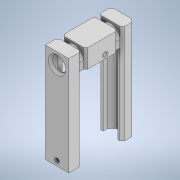
# Autodesk Inventor part: Magazin
Saved by Autodesk Inventor 2021 (Build 250183000, 183)
## iProperties
Created: 2024-05-14
Part Number: Magazin
Material: Generic
Document SubType Name: Modeling
Designer: Lukas
Density: 1 g/cm^3
Appearance: Default
Author: Lukas
Autodesk Inventor part; units mm, degrees
ref_plane "YZ Plane" through (0, 0, 0) normal (1, 0, 0) x (0, 1, 0)
ref_plane "XZ Plane" through (0, 0, 0) normal (0, 1, 0) x (-1, 0, 0)
ref_plane "XY Plane" through (0, 0, 0) normal (0, 0, 1) x (1, 0, 0)
sketch "Sketch1" plane through (0, 0, 0) normal (0, 0, 1) x (1, 0, 0)
  circle A0 centre (0, 0) radius 5
  line L0 (-8, 0) -> (-8, -60)
  line L1 (-8, -60) -> (8, -60)
  line L2 (8, -60) -> (8, 0)
  line L3 (8, 0) -> (8, 8)
  line L4 (8, 8) -> (-8, 8)
  line L5 (-8, 8) -> (-8, 0)
  point P0 (0, 8)
  dimension "d0" = 10
  dimension "d3" = 60
  dimension "d4" = 16
  dimension "d68" = 8
  constraints: 12 end point, 3 perpendicular, 2 horizontal alignment, 2 vertical, 1 centre point, 1 coincident, 1 collinear, 1 midpoint, 1 vertical alignment
  measures "d0" diameter of A0
  measures "d3" distance of L1.end L2.end
  measures "d4" distance between parallel lines of L2 L0
  measures "d68" distance of L4.end L0.start
extrude "Extrusion1" add sketch "Sketch1" along normal mid plane 45
sketch "Sketch3" plane through (-8, -60, -22.5) normal (0, -1, 0) x (1, 0, 0)
  line L0 (13, 45) -> (13, 0) projected
  line L1 (13, 5.5) -> (10, 2.5)
  line L2 (10, 2.5) -> (6, 2.5)
  line L3 (6, 2.5) -> (3, 5.5)
  line L4 (3, 45) -> (3, 0) projected
  line L5 (13, 39.5) -> (10, 42.5)
  line L6 (10, 42.5) -> (6, 42.5)
  line L7 (6, 42.5) -> (3, 39.5)
  line L8 (16, 0) -> (0, 0) projected
  point P0 (8, 22.5)
  point P1 (8, 0)
  dimension "d19" = 4
  dimension "d20" = 3
  dimension "d21" = 40
  dimension "d54" = 20
  constraints: 12 end point, 4 point on line, 3 equal length, 2 horizontal alignment, 2 parallel, 1 perpendicular, 2 other
  measures "d19" distance of L1.end L2.end
  measures "d20" distance from line of L2 L1.start
  measures "d21" distance between parallel lines of L2 L6
  measures "d54" distance from line of point (8, 22.5) L2
extrude "Extrusion3" cut sketch "Sketch3" against normal blind 60 contours L0 L1 L2 L3 L4 L7 L6 L5
sketch "Sketch4" plane through (-8, -60, -22.5) normal (0, -1, 0) x (1, 0, 0)
  line L0 (16, 0) -> (0, 0) projected
  line L1 (14.2, 0) -> (16, 1.8)
  line L2 (16, 0) -> (16, 45) projected
  line L3 (1.8, 0) -> (0, 1.8)
  line L4 (0, 0) -> (0, 45) projected
  line L5 (13, 5.5) -> (10, 2.5) projected
  point P0 (8, 22.5)
  dimension "d35" = 1.8
  constraints: 4 end point, 2 point on line, 1 horizontal alignment, 1 parallel, 1 perpendicular, 3 other
  measures "d35" horizontal distance of L1.start L1.end
extrude "Extrusion4" cut sketch "Sketch4" against normal through all
ref_plane "Work Plane3" through (0, 0, -2.4) normal (0, 0, 1) x (1, 0, 0)
sketch "Sketch5" plane through (0, 0, -2.4) normal (0, 0, 1) x (1, 0, 0)
  line L0 (8, -60) -> (8, 8) projected
  line L1 (8, -1) -> (8, -4)
  arc A0 (8, -1) -> (8, -4) centre (9.125, -2.5) ccw
  line L2 (9.125, -2.5) -> (9.125, -1.8268)
  point P0 (0, 0)
  point P1 (8, 0)
  point P2 (8, -1)
  dimension "d42" = 3
  dimension "d43" = 0.75
  dimension "d44" = 2.5
  dimension "d45" = 8
  constraints: 4 end point, 2 point on circle, 2 vertical, 1 centre point
  measures "d42" distance of L1.start L1.end
  measures "d43" distance edge to line of A0 L1
  measures "d44" vertical distance of point (0, 0) L2.start
  measures "d45" horizontal distance of point (0, 0) L1.start
revolve "Revolution1" cut sketch "Sketch5" angle 360 about axis through (9.125, -2.5, -2.4) along (0, 1, 0)
fillet "Fillet1" radius 1 2 edges at (8, -2.5, -0.9) (8, -2.5, -3.9)
mirror "Mirror1" about plane through (0, 0, 0) normal (1, 0, 0) of "Revolution1", "Fillet1"
ref_plane "Work Plane2" through (0, 0, -12.5) normal (0, 0, -1) x (-1, 0, 0)
sketch "Sketch6" plane through (0, 0, -12.5) normal (0, 0, -1) x (-1, 0, 0)
  line L0 (-8, -60) -> (-8, 8) projected
  line L1 (8, 8) -> (8, -60) projected
  arc A0 (6.5, 0) -> (-6.5, 0) centre (0, 0) ccw
  line L2 (6.5, 0) -> (6.5, -5)
  line L3 (6.5, -5) -> (5, -5)
  line L4 (5, -60) -> (5, 0) projected
  line L5 (-6.5, 0) -> (-6.5, -5)
  line L6 (-6.5, -5) -> (-5, -5)
  line L7 (-5, -60) -> (-5, 0) projected
  line L8 (8, -60) -> (-8, -60) projected
  line L9 (-8, 8) -> (8, 8) projected
  circle A1 centre (0, 0) radius 5 projected
  point P0 (-8, 0)
  point P1 (8, 0)
  dimension "d50" = 5
  dimension "d69" = 1.5
  constraints: 8 end point, 4 point on line, 2 perpendicular, 2 point on circle, 2 tangent, 1 centre point, 1 concentric, 1 vertical
  measures "d50" distance from line of point (0, 0) L6
  measures "d69" distance of L5.end L6.end
extrude "Extrusion5" cut sketch "Sketch6" against normal mid plane 3 contours L0 L9 L1 L8 L4 L3 L2 A0 L5 L6 L7
chamfer "Chamfer4" distance 1.5 angle 45 4 edges at (-8, -26, -11) (8, -26, -11) (-8, -26, -14) (8, -26, -14)
mirror "Mirror2" about plane through (0, 0, 0) normal (0, 0, 1) of "Extrusion5", "Chamfer4"
chamfer "Chamfer5" distance 1 distance2 2 1 edges at (-5, 0, 22.5) measured on face at (-5.5, 0, 22.5)
sketch "Sketch7" plane through (0, 0, 22.5) normal (0, 0, 1) x (1, 0, 0)
  circle A0 centre (0, -56.6) radius 1.6
  line L0 (-8, -60) -> (8, -60) projected
  point P0 (0, 0)
  point P1 (0, -60)
  dimension "d58" = 3.4
  dimension "d59" = 3.2
  constraints: 1 centre point, 1 midpoint, 1 vertical alignment
  measures "d58" distance from line of L0 A0.centre
  measures "d59" diameter of A0
extrude "Extrusion6" cut sketch "Sketch7" against normal through all
sketch "Sketch9" plane through (-6.5, -60, -11) normal (0, -1, 0) x (1, 0, 0)
  line L0 (13, 22) -> (14.5, 20.5) projected
  line L1 (13, 22) -> (11.5, 22) projected
  line L2 (11.5, 22) -> (11.5, 0) projected
  line L3 (11.5, 0) -> (13, 0) projected
  line L4 (14.5, 1.5) -> (13, 0) projected
  line L5 (14.5, 1.5) -> (14.5, 20.5) projected
  line L6 (-1.5, 20.5) -> (0, 22) projected
  line L7 (-1.5, 1.5) -> (-1.5, 20.5) projected
  line L8 (0, 0) -> (-1.5, 1.5) projected
  line L9 (0, 0) -> (1.5, 0) projected
  line L10 (1.5, 0) -> (1.5, 22) projected
  line L11 (1.5, 22) -> (0, 22) projected
  point P0 (6.5, 11)
extrude "Extrusion8" cut sketch "Sketch9" against normal up to surface (55 mm away)
move faces "Move1" translate (0, -0.25, 0) faces at (2.1667, 8, 19.6667) (2.6667, 8, -3.1667) (2.0667, 8, -16.8333)
equation "\"d54\" = 0.5 * d21"
body "Solid1"
